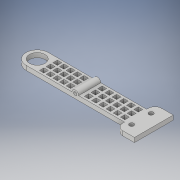
# Autodesk Inventor part: Side V2
Saved by Autodesk Inventor 2019 (Build 230136000, 136)
## iProperties
Created: 2018-11-04
Part Number: Side V2
Material: Generic
Document SubType Name: Modeling
Designer: mrhftc
Density: 1 g/cm^3
Appearance: Default
Author: mrhftc
Autodesk Inventor part; units mm, degrees
ref_plane "YZ Plane" through (0, 0, 0) normal (1, 0, 0) x (0, 1, 0)
ref_plane "XZ Plane" through (0, 0, 0) normal (0, 1, 0) x (-1, 0, 0)
ref_plane "XY Plane" through (0, 0, 0) normal (0, 0, 1) x (1, 0, 0)
sketch "Main Sketch" plane through (0, 0, 0) normal (0, 1, 0) x (-1, 0, 0)
  line L0 (-57.375, -12.0472) -> (-57.375, 12.0472)
  line L1 (-57.375, 12.0472) -> (47.625, -10) construction
  line L2 (47.625, 10) -> (-57.375, -12.0472) construction
  circle A0 centre (47.625, 0) radius 7
  arc A1 (47.625, -10) -> (47.625, 10) centre (47.625, 0) ccw
  line L3 (-40.875, 17.5) -> (-57.375, 17.5)
  line L4 (-57.375, 17.5) -> (-57.375, -17.5)
  line L5 (-57.375, -17.5) -> (-40.875, -17.5)
  line L6 (-40.875, 17.5) -> (-57.375, -17.5) construction
  line L7 (-57.375, 17.5) -> (-40.875, -17.5) construction
  line L8 (47.625, -10) -> (-40.875, -10)
  line L9 (-40.875, -17.5) -> (-40.875, -10)
  line L10 (-40.875, 10) -> (-40.875, 17.5)
  line L11 (-40.875, 10) -> (47.625, 10)
  point P0 (0, 0)
  point P1 (-49.125, 0)
  dimension "d3" = 14
  dimension "d4" = 105
  dimension "d13" = 16.5
  dimension "d14" = 35
  dimension "d15" = 0
  dimension "d18" = 20
  constraints: 24 end point, 4 parallel, 2 centre point, 2 horizontal, 2 midpoint, 2 point on circle, 2 point on line, 1 coincident, 1 perpendicular
  measures "d3" diameter of A0
  measures "d4" distance from line of L0 A0.centre
  measures "d13" distance of L4.end L5.end
  measures "d14" distance of L3.end L4.end
  measures "d15" distance between parallel lines of L0 L4
  measures "d18" distance between parallel lines of L11 L8
extrude "Main Extrusion" add sketch "Main Sketch" along normal blind 4
sketch "Screw Holes Sketch" plane through (0, 4, 0) normal (0, 1, 0) x (1, 0, 0)
  circle A0 centre (46.125, -8.75) radius 2
  line L0 (57.375, 17.5) -> (40.875, 17.5) projected
  line L1 (40.875, -17.5) -> (57.375, -17.5) projected
  line L2 (35.2664, 0) -> (65.7891, 0)
  line L3 (51.375, -27.0398) -> (51.375, 30.2346) construction
  line L4 (57.375, -17.5) -> (57.375, 17.5) projected
  line L5 (40.875, -10) -> (40.875, -17.5) projected
  circle A1 centre (46.125, 8.75) radius 2
  line L6 (51.375, 27.0398) -> (51.375, -30.2346) construction
  point P0 (0, 0)
  dimension "d21" = 4
  dimension "d22" = 35
  dimension "d23" = 6
  dimension "d24" = 5.25
  dimension "d25" = 5.25
  dimension "d26" = 10.5
  dimension "d27" = 8.75
  dimension "d28" = 17.5
  constraints: 6 end point, 3 symmetric about line, 2 centre point, 1 horizontal, 1 vertical, 1 other
  measures "d21" diameter of A0
  measures "d22" distance between parallel lines of L0 L1
  measures "d23" distance between parallel lines of L4 L3
  measures "d24" distance from line of L3 A0.centre
  measures "d25" distance from line of L5 A0.centre
  measures "d26" distance between parallel lines of L3 L5
  measures "d27" distance from line of L1 A0.centre
  measures "d28" diameter of A0.centre L2
extrude "Screw Holes Cut" cut sketch "Screw Holes Sketch" against normal through all
fillet "Smoooooooooooooooooth" radius 6 2 edges at (40.875, 2, -17.5) (40.875, 2, 17.5)
sketch "Side Axel Hole Sketch" plane through (-47.625, 0, 10) normal (0, 0, 1) x (1, 0, 0)
  line L0 (88.5, 4) -> (88.5, 0) projected
  line L1 (0, 0) -> (0, 4) projected
  line L2 (44.25, -12.0383) -> (44.25, 22.7681) construction
  line L3 (88.5, 0) -> (0, 0) projected
  line L4 (0, 4) -> (88.5, 4) projected
  circle A0 centre (44.25, 4) radius 1.5
  point P0 (47.625, 0)
  dimension "d32" = 88.5
  dimension "d33" = 44.25
  dimension "d34" = 44.25
  dimension "d35" = 4
  dimension "d41" = 3
  constraints: 2 end point, 1 centre point, 1 midpoint, 1 vertical
  measures "d32" distance between parallel lines of L0 L1
  measures "d33" distance between parallel lines of L1 L2
  measures "d34" distance between parallel lines of L0 L2
  measures "d35" distance between parallel lines of L3 L4
  measures "d41" diameter of A0
extrude "Side Axel Hole Cut" cut sketch "Side Axel Hole Sketch" against normal blind 20 contours A0 L4 | L4 A0
sketch "Side Hole Extension Sketch" plane through (-47.625, 0, 10) normal (0, 0, 1) x (1, 0, 0)
  arc A0 (42.75, 4) -> (45.75, 4) centre (44.25, 4) ccw projected
  circle A1 centre (44.25, 4) radius 3
  circle A2 centre (44.25, 4) radius 1.5
  point P0 (47.625, 0)
  dimension "d44" = 6
  constraints: 2 centre point, 2 coincident, 1 concentric
  measures "d44" diameter of A1
extrude "Extrusion7" add sketch "Side Hole Extension Sketch" against normal blind 20
sketch "Sketch7" plane through (0, 4, 0) normal (0, 1, 0) x (1, 0, 0)
  line L0 (-37.5494, 8) -> (-33.5494, 8)
  line L1 (-33.5494, 8) -> (-33.5494, 4)
  line L2 (-33.5494, 4) -> (-37.5494, 4)
  line L3 (-37.5494, 4) -> (-37.5494, 8)
  line L4 (-6.375, 10) -> (-47.625, 10) projected
  line L5 (-61.0525, 0) -> (64.9416, 0) construction
  line L6 (0, 19.4687) -> (0, -18.1059) construction
  line L7 (-47.5494, 9.1434) -> (-47.5494, -10.5737) construction
  line L8 (-37.5494, 2) -> (-33.5494, 2)
  line L9 (-33.5494, 2) -> (-33.5494, -2)
  line L10 (-33.5494, -2) -> (-37.5494, -2)
  line L11 (-37.5494, -2) -> (-37.5494, 2)
  line L12 (-37.5494, -4) -> (-33.5494, -4)
  line L13 (-33.5494, -4) -> (-33.5494, -8)
  line L14 (-33.5494, -8) -> (-37.5494, -8)
  line L15 (-37.5494, -8) -> (-37.5494, -4)
  line L16 (-31.5494, 8) -> (-27.5494, 8)
  line L17 (-27.5494, 8) -> (-27.5494, 4)
  line L18 (-27.5494, 4) -> (-31.5494, 4)
  line L19 (-31.5494, 4) -> (-31.5494, 8)
  line L20 (-31.5494, 2) -> (-27.5494, 2)
  line L21 (-27.5494, 2) -> (-27.5494, -2)
  line L22 (-27.5494, -2) -> (-31.5494, -2)
  line L23 (-31.5494, -2) -> (-31.5494, 2)
  line L24 (-31.5494, -4) -> (-27.5494, -4)
  line L25 (-27.5494, -4) -> (-27.5494, -8)
  line L26 (-27.5494, -8) -> (-31.5494, -8)
  line L27 (-31.5494, -8) -> (-31.5494, -4)
  line L28 (-25.5494, 8) -> (-21.5494, 8)
  line L29 (-21.5494, 8) -> (-21.5494, 4)
  line L30 (-21.5494, 4) -> (-25.5494, 4)
  line L31 (-25.5494, 4) -> (-25.5494, 8)
  line L32 (-25.5494, 2) -> (-21.5494, 2)
  line L33 (-21.5494, 2) -> (-21.5494, -2)
  line L34 (-21.5494, -2) -> (-25.5494, -2)
  line L35 (-25.5494, -2) -> (-25.5494, 2)
  line L36 (-25.5494, -4) -> (-21.5494, -4)
  line L37 (-21.5494, -4) -> (-21.5494, -8)
  line L38 (-21.5494, -8) -> (-25.5494, -8)
  line L39 (-25.5494, -8) -> (-25.5494, -4)
  line L40 (-19.5494, 8) -> (-15.5494, 8)
  line L41 (-15.5494, 8) -> (-15.5494, 4)
  line L42 (-15.5494, 4) -> (-19.5494, 4)
  line L43 (-19.5494, 4) -> (-19.5494, 8)
  line L44 (-19.5494, 2) -> (-15.5494, 2)
  line L45 (-15.5494, 2) -> (-15.5494, -2)
  line L46 (-15.5494, -2) -> (-19.5494, -2)
  line L47 (-19.5494, -2) -> (-19.5494, 2)
  line L48 (-19.5494, -4) -> (-15.5494, -4)
  line L49 (-15.5494, -4) -> (-15.5494, -8)
  line L50 (-15.5494, -8) -> (-19.5494, -8)
  line L51 (-19.5494, -8) -> (-19.5494, -4)
  line L52 (-13.5494, 8) -> (-9.5494, 8)
  line L53 (-9.5494, 8) -> (-9.5494, 4)
  line L54 (-9.5494, 4) -> (-13.5494, 4)
  line L55 (-13.5494, 4) -> (-13.5494, 8)
  line L56 (-13.5494, 2) -> (-9.5494, 2)
  line L57 (-9.5494, 2) -> (-9.5494, -2)
  line L58 (-9.5494, -2) -> (-13.5494, -2)
  line L59 (-13.5494, -2) -> (-13.5494, 2)
  line L60 (-13.5494, -4) -> (-9.5494, -4)
  line L61 (-9.5494, -4) -> (-9.5494, -8)
  line L62 (-9.5494, -8) -> (-13.5494, -8)
  line L63 (-13.5494, -8) -> (-13.5494, -4)
  line L64 (-47.625, -10) -> (-6.375, -10) projected
  line L65 (2.7994, 8) -> (6.7994, 8)
  line L66 (6.7994, 8) -> (6.7994, 4)
  line L67 (6.7994, 4) -> (2.7994, 4)
  line L68 (2.7994, 4) -> (2.7994, 8)
  line L69 (40.875, 10) -> (-0.375, 10) projected
  line L70 (-6.375, -10) -> (-6.375, 10) projected
  line L71 (-0.375, 10) -> (-0.375, -10) projected
  line L72 (6.7994, -2) -> (2.7994, -2)
  line L73 (2.7994, 2) -> (6.7994, 2)
  line L74 (6.7994, 2) -> (6.7994, -2)
  line L75 (2.7994, -2) -> (2.7994, 2)
  line L76 (0, 13.4687) -> (0, -24.1059) construction
  line L77 (6.7994, -8) -> (2.7994, -8)
  line L78 (2.7994, -4) -> (6.7994, -4)
  line L79 (6.7994, -4) -> (6.7994, -8)
  line L80 (2.7994, -8) -> (2.7994, -4)
  line L81 (0, 7.4687) -> (0, -30.1059) construction
  line L82 (13.2994, 4) -> (9.2994, 4)
  line L83 (9.2994, 8) -> (13.2994, 8)
  line L84 (13.2994, 8) -> (13.2994, 4)
  line L85 (9.2994, 4) -> (9.2994, 8)
  line L86 (6.5, 19.4687) -> (6.5, -18.1059) construction
  line L87 (13.2994, -2) -> (9.2994, -2)
  line L88 (9.2994, 2) -> (13.2994, 2)
  line L89 (13.2994, 2) -> (13.2994, -2)
  line L90 (9.2994, -2) -> (9.2994, 2)
  line L91 (6.5, 13.4687) -> (6.5, -24.1059) construction
  line L92 (13.2994, -8) -> (9.2994, -8)
  line L93 (9.2994, -4) -> (13.2994, -4)
  line L94 (13.2994, -4) -> (13.2994, -8)
  line L95 (9.2994, -8) -> (9.2994, -4)
  line L96 (6.5, 7.4687) -> (6.5, -30.1059) construction
  line L97 (19.7994, 4) -> (15.7994, 4)
  line L98 (15.7994, 8) -> (19.7994, 8)
  line L99 (19.7994, 8) -> (19.7994, 4)
  line L100 (15.7994, 4) -> (15.7994, 8)
  line L101 (13, 19.4687) -> (13, -18.1059) construction
  line L102 (19.7994, -2) -> (15.7994, -2)
  line L103 (15.7994, 2) -> (19.7994, 2)
  line L104 (19.7994, 2) -> (19.7994, -2)
  line L105 (15.7994, -2) -> (15.7994, 2)
  line L106 (13, 13.4687) -> (13, -24.1059) construction
  line L107 (19.7994, -8) -> (15.7994, -8)
  line L108 (15.7994, -4) -> (19.7994, -4)
  line L109 (19.7994, -4) -> (19.7994, -8)
  line L110 (15.7994, -8) -> (15.7994, -4)
  line L111 (13, 7.4687) -> (13, -30.1059) construction
  line L112 (26.2994, 4) -> (22.2994, 4)
  line L113 (22.2994, 8) -> (26.2994, 8)
  line L114 (26.2994, 8) -> (26.2994, 4)
  line L115 (22.2994, 4) -> (22.2994, 8)
  line L116 (19.5, 19.4687) -> (19.5, -18.1059) construction
  line L117 (26.2994, -2) -> (22.2994, -2)
  line L118 (22.2994, 2) -> (26.2994, 2)
  line L119 (26.2994, 2) -> (26.2994, -2)
  line L120 (22.2994, -2) -> (22.2994, 2)
  line L121 (19.5, 13.4687) -> (19.5, -24.1059) construction
  line L122 (26.2994, -8) -> (22.2994, -8)
  line L123 (22.2994, -4) -> (26.2994, -4)
  line L124 (26.2994, -4) -> (26.2994, -8)
  line L125 (22.2994, -8) -> (22.2994, -4)
  line L126 (19.5, 7.4687) -> (19.5, -30.1059) construction
  line L127 (32.7994, 4) -> (28.7994, 4)
  line L128 (28.7994, 8) -> (32.7994, 8)
  line L129 (32.7994, 8) -> (32.7994, 4)
  line L130 (28.7994, 4) -> (28.7994, 8)
  line L131 (26, 19.4687) -> (26, -18.1059) construction
  line L132 (32.7994, -2) -> (28.7994, -2)
  line L133 (28.7994, 2) -> (32.7994, 2)
  line L134 (32.7994, 2) -> (32.7994, -2)
  line L135 (28.7994, -2) -> (28.7994, 2)
  line L136 (26, 13.4687) -> (26, -24.1059) construction
  line L137 (32.7994, -8) -> (28.7994, -8)
  line L138 (28.7994, -4) -> (32.7994, -4)
  line L139 (32.7994, -4) -> (32.7994, -8)
  line L140 (28.7994, -8) -> (28.7994, -4)
  line L141 (26, 7.4687) -> (26, -30.1059) construction
  line L142 (39.2994, 4) -> (35.2994, 4)
  line L143 (35.2994, 8) -> (39.2994, 8)
  line L144 (39.2994, 8) -> (39.2994, 4)
  line L145 (35.2994, 4) -> (35.2994, 8)
  line L146 (32.5, 19.4687) -> (32.5, -18.1059) construction
  line L147 (39.2994, -2) -> (35.2994, -2)
  line L148 (35.2994, 2) -> (39.2994, 2)
  line L149 (39.2994, 2) -> (39.2994, -2)
  line L150 (35.2994, -2) -> (35.2994, 2)
  line L151 (32.5, 13.4687) -> (32.5, -24.1059) construction
  line L152 (39.2994, -8) -> (35.2994, -8)
  line L153 (35.2994, -4) -> (39.2994, -4)
  line L154 (39.2994, -4) -> (39.2994, -8)
  line L155 (35.2994, -8) -> (35.2994, -4)
  line L156 (32.5, 7.4687) -> (32.5, -30.1059) construction
  point P0 (0, 0)
  point P1 (-47.625, 0)
  dimension "d47" = 4
  dimension "d48" = 4
  dimension "d49" = 2
  dimension "d52" = 10
  dimension "d55" = 6
  dimension "d58" = 6
  dimension "d61" = 2
  dimension "d62" = 4
  dimension "d63" = 4
  dimension "d64" = 2
  dimension "d65" = 3.1744
  dimension "d66" = 3.1744
  dimension "d69" = 6
  dimension "d72" = 6.5
  constraints: 304 end point, 5 horizontal, 4 parallel, 4 vertical, 2 perpendicular, 1 collinear, 1 point on line, 298 other
  measures "d47" distance of L0.start L0.end
  measures "d48" distance of L0.end L1.end
  measures "d49" distance between parallel lines of L4 L0
  measures "d52" distance between parallel lines of L3 L7
  measures "d55" distance of L0.start L8.start
  measures "d58" distance of L0.start L16.start
  measures "d61" distance between parallel lines of L64 L14
  measures "d62" distance of L65.start L65.end
  measures "d63" distance of L65.end L66.end
  measures "d64" distance between parallel lines of L69 L65
  measures "d65" distance between parallel lines of L70 L53
  measures "d66" distance between parallel lines of L68 L71
  measures "d69" distance of L67.end L72.end
  measures "d72" distance of L67.end L82.end
extrude "Extrusion8" cut sketch "Sketch7" against normal through all
body "Solid3"
